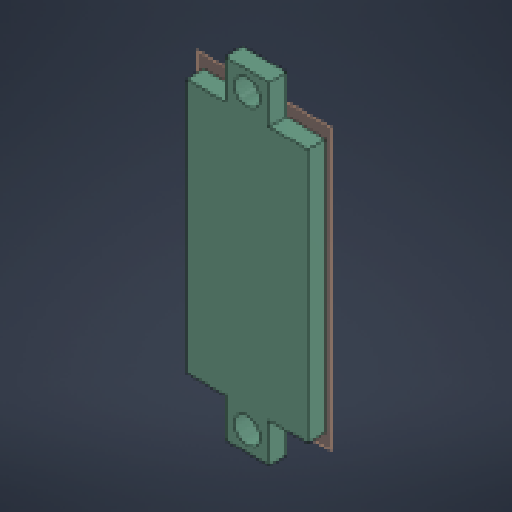
# Autodesk Inventor part: Segment_PCB
Saved by Autodesk Inventor 2024.2 (Build 282272000, 272)
## iProperties
Created: 2024-01-12
Part Number: Segment_PCB
Material: 一般
Document SubType Name: Modeling
Designer: Hanaoka
Density: 1 g/cm^3
Appearance: 既定
Author: Hanaoka
Autodesk Inventor part; units mm, degrees
ref_plane "YZ Plane" through (0, 0, 0) normal (1, 0, 0) x (0, 1, 0)
ref_plane "XZ Plane" through (0, 0, 0) normal (0, 1, 0) x (-1, 0, 0)
ref_plane "XY Plane" through (0, 0, 0) normal (0, 0, 1) x (1, 0, 0)
ref_plane "作業平面1" through (0, 0, 0) normal (0, 0, 1) x (1, 0, 0)
sketch "スケッチ1" plane through (0, 0, 0) normal (0, 0, 1) x (1, 0, 0)
  line L0 (5.5, -11.5) -> (-5.5, -11.5) projected
  line L1 (5.5, 11.5) -> (5.5, -11.5) projected
  line L2 (-5.5, 11.5) -> (5.5, 11.5) projected
  line L3 (-5.5, -11.5) -> (-5.5, 11.5) projected
  line L4 (2, 11.5) -> (-2, 11.5)
  line L5 (-2, 11.5) -> (-2, 15)
  line L6 (-2, 15) -> (2, 15)
  line L7 (2, 15) -> (2, 11.5)
  line L8 (2, -11.5) -> (-2, -11.5)
  line L9 (-2, -11.5) -> (-2, -15)
  line L10 (-2, -15) -> (2, -15)
  line L11 (2, -15) -> (2, -11.5)
  line L12 (0, -21) -> (0, 21) projected
  circle A0 centre (0, 13.25) radius 1.15
  circle A1 centre (0, -13.25) radius 1.15
  line L13 (2, 13.25) -> (-2, 13.25) construction
  line L14 (2, -13.25) -> (-2, -13.25) construction
  point P0 (0, 0)
  point P1 (0, 15)
  dimension "d0" = 3.5
  dimension "d1" = 4
  dimension "d2" = 2.3
  constraints: 20 end point, 7 midpoint, 7 point on line, 4 parallel, 2 centre point, 2 horizontal, 2 perpendicular, 1 collinear, 1 equal radius
  measures "d0" distance of L10.end L8.start
  measures "d1" distance of L9.end L10.end
  measures "d2" diameter of A0
extrude "押し出し1" add sketch "スケッチ1" along normal blind 1.6 contours L0 L12 L2 L1 | L11 L10 L12 A1 L0 | L12 A1 L10 L9 L0 | L0 L3 L2 L12 | L2 L12 A0 L6 L7 | L2 L5 L6 L12 A0
